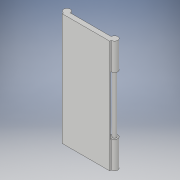
# Autodesk Inventor part: leftRightPlate
Saved by Autodesk Inventor 2019 (Build 230136000, 136)
## iProperties
Created: 2018-07-23
Part Number: leftRightPlate
Material: Generic
Document SubType Name: Modeling
Designer: Ge Shi
Density: 1 g/cm^3
Appearance: Default
Author: Ge Shi
Autodesk Inventor part; units mm, degrees
ref_plane "YZ Plane" through (0, 0, 0) normal (1, 0, 0) x (0, 1, 0)
ref_plane "XZ Plane" through (0, 0, 0) normal (0, 1, 0) x (-1, 0, 0)
ref_plane "XY Plane" through (0, 0, 0) normal (0, 0, 1) x (1, 0, 0)
sketch "Sketch1" plane through (0, 0, 0) normal (0, 0, 1) x (1, 0, 0)
  line L0 (20, -47.25) -> (-20, -47.25)
  line L1 (-20, -47.25) -> (-20, 47.25)
  line L2 (-20, 47.25) -> (20, 47.25)
  line L3 (20, 47.25) -> (20, -47.25)
  line L4 (20, -47.25) -> (-20, 47.25) construction
  line L5 (-20, -47.25) -> (20, 47.25) construction
  point P0 (0, 0)
  dimension "d0" = 40
  dimension "d1" = 94.5
  constraints: 12 end point, 2 midpoint, 2 parallel, 1 horizontal, 1 perpendicular
  measures "d0" distance of L1.end L2.end
  measures "d1" distance of L0.end L1.end
extrude "Extrusion1" add sketch "Sketch1" along normal blind 4
ref_plane "Work Plane1" through (-20, 0, 0) normal (0, 1, 0) x (1, 0, 0)
sketch "Sketch2" plane through (-20, 0, 0) normal (0, 1, 0) x (1, 0, 0)
  circle A0 centre (0, 0) radius 1.5
  circle A1 centre (40, 0) radius 1.5
  circle A2 centre (0, 0) radius 2.75
  circle A3 centre (40, 0) radius 2.75
  line L0 (40, 0) -> (0, 0) projected
  circle A4 centre (0, 0) radius 3.5
  circle A5 centre (40, 0) radius 3.5
  point P0 (20, 0)
  dimension "d4" = 3
  dimension "d5" = 3
  dimension "d6" = 5.5
  dimension "d7" = 5.5
  dimension "d14" = 7
  dimension "d15" = 7
  constraints: 6 centre point, 4 coincident
  measures "d4" diameter of A0
  measures "d5" diameter of A1
  measures "d6" diameter of A2
  measures "d7" diameter of A3
  measures "d14" diameter of A4
  measures "d15" diameter of A5
extrude "Extrusion2" cut sketch "Sketch2" along normal mid plane 94.5 contours A0 | A1 | A2 | A3
extrude "Extrusion3" add sketch "Sketch2" along normal mid plane 94.5 contours A2 | A3
extrude "Extrusion4" cut sketch "Sketch2" along normal mid plane 48.75 contours A2 | A3 | A4 | A5
extrude "Extrusion5" add sketch "Sketch2" along normal mid plane 94.5 contours A0 | A1
chamfer "Chamfer2" distance 1.5 angle 45 1 edges at (-21.9445, -47.25, -1.9445)
equation "\"d0\" = width"
equation "\"d1\" = height - hingeShaftHolder"
equation "\"d2\" = thick"
equation "\"d4\" = hingeShaft"
equation "\"d5\" = hingeShaft"
equation "\"d6\" = hingeShaftHolder"
equation "\"d7\" = hingeShaftHolder"
equation "\"d14\" = hingeShaftHolder + clearance"
equation "\"d15\" = hingeShaftHolder + clearance"
equation "\"d8\" = height - hingeShaftHolder"
equation "\"d10\" = height - hingeShaftHolder"
equation "\"d16\" = height - hingeShaftHolder"
equation "\"width\" = 40"
equation "\"height\" = 100"
equation "\"hingeShaftHolder\" = 5.5"
equation "\"thick\" = 4"
equation "\"hingeShaft\" = 3"
equation "\"clearance\" = 1.5"
body "Solid1"
